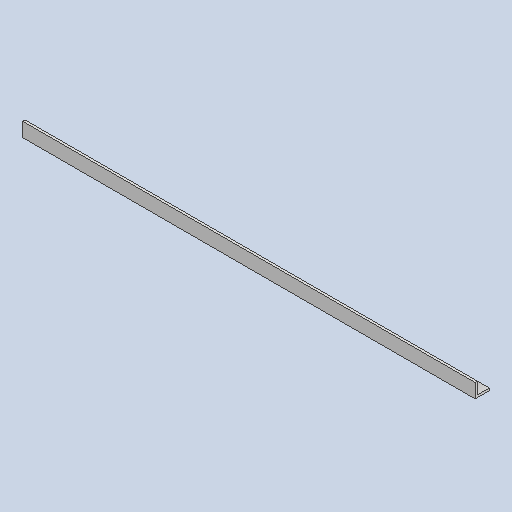
# Autodesk Inventor part: LatL24T
Saved by Autodesk Inventor 2023 (Build 270158030, 158C)
## iProperties
Created: 2022-07-27
Part Number: LatL24T
Material: Generic
Document SubType Name: Modeling
Designer: jeremyy
Density: 1 g/cm^3
Appearance: Default
Author: jeremyy
Autodesk Inventor part; units mm, degrees
ref_plane "YZ Plane" through (0, 0, 0) normal (1, 0, 0) x (0, 1, 0)
ref_plane "XZ Plane" through (0, 0, 0) normal (0, 1, 0) x (-1, 0, 0)
ref_plane "XY Plane" through (0, 0, 0) normal (0, 0, 1) x (1, 0, 0)
sketch "Sketch1" plane through (0, 0, 0) normal (1, 0, 0) x (0, 1, 0)
  line L0 (0, 0) -> (0, -19.05)
  line L1 (0, -19.05) -> (3.175, -19.05)
  line L2 (3.175, -19.05) -> (3.175, -3.175)
  line L3 (3.175, -3.175) -> (19.05, -3.175)
  line L4 (19.05, -3.175) -> (19.05, 0)
  line L5 (19.05, 0) -> (0, 0)
  dimension "d0" = 19.05
  dimension "d1" = 3.175
  dimension "d2" = 15.875
  dimension "d3" = 15.875
  constraints: 12 end point, 5 perpendicular, 1 vertical
  measures "d0" distance of L0.start L0.end
  measures "d1" distance of L0.end L1.end
  measures "d2" distance of L1.end L2.end
  measures "d3" distance of L2.end L3.end
extrude "Extrusion1" add sketch "Sketch1" along normal blind 609.6
body "Solid1"
